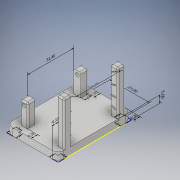
# Autodesk Inventor part: FanTable
Saved by Autodesk Inventor 2019 (Build 230136000, 136)
## iProperties
Created: 2018-06-07
Part Number: FanTable
Material: Ogólny
Document SubType Name: Modeling
Designer: Kamil
Density: 1 g/cm^3
Appearance: Domyślna
Author: Kamil
## iProperties of the stored document FanTable_Drukowanie 3D.ipt
Created: 2018-06-18
Part Number: FanTable_Drukowanie 3D
Material: Ogólny
Document SubType Name: Modeling
Designer: Kamil
Density: 1 g/cm^3
Appearance: Domyślna
Author: Kamil
Autodesk Inventor part; units mm, degrees
ref_plane "YZ Plane" through (0, 0, 0) normal (1, 0, 0) x (0, 1, 0)
ref_plane "XZ Plane" through (0, 0, 0) normal (0, 1, 0) x (-1, 0, 0)
ref_plane "XY Plane" through (0, 0, 0) normal (0, 0, 1) x (1, 0, 0)
sketch "Szkic1" plane through (0, 0, 0) normal (0, 1, 0) x (-1, 0, 0)
  line L0 (-17, -25) -> (18, -25)
  line L1 (18, -25) -> (18, 25)
  line L2 (18, 25) -> (-17, 25)
  line L3 (-17, 25) -> (-17, -25)
  dimension "d2" = 35
  dimension "d3" = 50
  constraints: 8 end point, 2 parallel, 1 horizontal, 1 perpendicular
  measures "d2" distance of L2.end L1.end
  measures "d3" distance of L1.end L0.end
extrude "Wyciągnięcie proste1" add sketch "Szkic1" along normal blind 5
sketch "Szkic2" plane through (0, 0, 0) normal (0, -1, 0) x (1, 0, 0)
  line L0 (17, 25) -> (17, -25) projected
  line L1 (17, 25) -> (13, 25)
  line L2 (13, 25) -> (13, 21)
  line L3 (13, 21) -> (17, 21)
  line L4 (17, 21) -> (17, 25)
  line L5 (-18, -25) -> (-18, 25) projected
  line L6 (-18, 25) -> (-14, 25)
  line L7 (-14, 25) -> (-14, 21)
  line L8 (-14, 21) -> (-18, 21)
  line L9 (-18, 21) -> (-18, 25)
  line L10 (17, -25) -> (-18, -25) projected
  line L11 (-18, -25) -> (-14, -25)
  line L12 (-14, -25) -> (-14, -21)
  line L13 (-14, -21) -> (-18, -21)
  line L14 (-18, -21) -> (-18, -25)
  line L15 (17, -25) -> (13, -25)
  line L16 (13, -25) -> (13, -21)
  line L17 (13, -21) -> (17, -21)
  line L18 (17, -21) -> (17, -25)
  point P0 (0, 0)
  dimension "d6" = 4
  dimension "d7" = 4
  dimension "d8" = 4
  dimension "d9" = 4
  dimension "d10" = 4
  dimension "d11" = 4
  dimension "d12" = 4
  constraints: 32 end point, 8 parallel, 4 horizontal, 4 perpendicular
  measures "d6" distance of L3.end L2.end
  measures "d7" distance of L2.end L1.end
  measures "d8" distance of L7.end L8.end
  measures "d9" distance of L6.end L7.end
  measures "d10" distance of L12.end L11.end
  measures "d11" distance of L16.end L17.end
  measures "d12" distance of L15.end L16.end
sketch "Szkic3" plane through (17, 0, 25) normal (1, 0, 0) x (0, 0, -1)
  point P0 (25, 0)
sketch "Szkic4" plane through (0, 0, 0) normal (0, -1, 0) x (1, 0, 0)
  point P0 (0, 0)
sketch "Szkic5" plane through (-18, 0, 25) normal (-1, 0, 0) x (0, 0, 1)
  point P0 (-25, 0)
fillet "Zaokrąglenie2" radius 4 1 edges at (17, 2.5, 25)
fillet "Zaokrąglenie4" radius 4 1 edges at (17, 2.5, -25)
fillet "Zaokrąglenie6" radius 4 1 edges at (-18, 2.5, 25)
fillet "Zaokrąglenie8" radius 4 1 edges at (-18, 2.5, -25)
sketch "Szkic7" plane through (0, 5, 0) normal (0, 1, 0) x (1, 0, 0)
  line L0 (-13, 15.7) -> (-8, 15.7)
  line L1 (-8, 15.7) -> (-8, 20.7)
  line L2 (-8, 20.7) -> (-13, 20.7)
  line L3 (-13, 20.7) -> (-13, 15.7)
  line L4 (-13, -15.7) -> (-8, -15.7)
  line L5 (-8, -15.7) -> (-8, -20.7)
  line L6 (-8, -20.7) -> (-13, -20.7)
  line L7 (-13, -20.7) -> (-13, -15.7)
  point P0 (0, 0)
  dimension "d114" = 1.5
  dimension "d31" = 5
  dimension "d32" = 5
  dimension "d33" = 5
  dimension "d34" = 5
  constraints: 16 end point, 4 parallel, 2 horizontal, 2 perpendicular
  measures "d31" distance of L2.end L1.end
  measures "d32" distance of L1.end L0.end
  measures "d33" distance of L5.end L6.end
  measures "d34" distance of L4.end L5.end
extrude "Wyciągnięcie proste4" add sketch "Szkic7" along normal blind 15
sketch "Szkic8" plane through (-13, 5, -15.7) normal (0, 0, 1) x (1, 0, 0)
  circle A0 centre (2.5, 12.5) radius 1.25
  point P0 (13, -5)
  dimension "d37" = 2.5
  constraints: 1 centre point
  measures "d37" diameter of A0
sketch "Szkic9" plane through (-8, 5, 15.7) normal (0, 0, -1) x (-1, 0, 0)
  circle A0 centre (2.5, 12.5) radius 1.25
  point P0 (-8, -5)
  dimension "d159" = 2.5
  constraints: 1 centre point
  measures "d159" diameter of A0
fillet "Zaokrąglenie9" radius 1 1 edges at (-13, 20, -18.2)
fillet "Zaokrąglenie10" radius 1 3 edges at (-10, 20, -20.7) (-12.7071, 19.7071, -20.7) (-13, 12, -20.7)
fillet "Zaokrąglenie11" radius 1 3 edges at (-8, 20, -17.7) (-8, 19.7071, -20.4071) (-8, 12, -20.7)
fillet "Zaokrąglenie12" radius 1 1 edges at (-13, 20, 18.2)
fillet "Zaokrąglenie13" radius 1 3 edges at (-10, 20, 20.7) (-12.7071, 19.7071, 20.7) (-13, 12, 20.7)
fillet "Zaokrąglenie14" radius 1 3 edges at (-8, 20, 17.7) (-8, 19.7071, 20.4071) (-8, 12, 20.7)
sketch "Szkic10" plane through (0, 5, 0) normal (0, 1, 0) x (1, 0, 0)
  line L0 (17, -21) -> (17, 21) projected
  line L1 (17, 15.7) -> (12, 15.7)
  line L2 (12, 15.7) -> (12, 20.7)
  line L3 (12, 20.7) -> (17, 20.7)
  line L4 (17, 20.7) -> (17, 15.7)
  line L5 (17, -15) -> (12, -15)
  line L6 (12, -15) -> (12, -20)
  line L7 (12, -20) -> (17, -20)
  line L8 (17, -20) -> (17, -15)
  point P0 (0, 0)
  dimension "d57" = 5
  dimension "d58" = 5
  dimension "d59" = 5
  dimension "d60" = 5
  constraints: 16 end point, 4 parallel, 2 horizontal, 2 perpendicular, 2 point on line
  measures "d57" distance of L2.end L3.end
  measures "d58" distance of L1.end L2.end
  measures "d59" distance of L7.end L6.end
  measures "d60" distance of L6.end L5.end
extrude "Wyciągnięcie proste7" add sketch "Szkic10" along normal blind 15 contours L1 L2 L3 L0
sketch "Szkic11" plane through (0, 5, 0) normal (0, 1, 0) x (1, 0, 0)
  line L0 (17, -21) -> (17, 21) projected
  line L1 (17, -15.7) -> (12, -15.7)
  line L2 (12, -15.7) -> (12, -20.7)
  line L3 (12, -20.7) -> (17, -20.7)
  line L4 (17, -20.7) -> (17, -15.7)
  point P0 (0, 0)
  dimension "d63" = 5
  dimension "d64" = 5
  constraints: 8 end point, 2 parallel, 1 horizontal, 1 perpendicular, 1 point on line
  measures "d63" distance of L3.end L2.end
  measures "d64" distance of L2.end L1.end
extrude "Wyciągnięcie proste8" add sketch "Szkic11" along normal blind 15
sketch "Szkic15" plane through (0, 20, 0) normal (0, 1, 0) x (1, 0, 0)
  line L0 (12, 15.7) -> (12, 20.7) projected
  line L1 (12, 20.7) -> (17, 20.7)
  line L2 (17, 20.7) -> (17, 15.7)
  line L3 (17, 15.7) -> (12, 15.7)
  line L4 (12, 15.7) -> (12, 20.7)
  line L5 (17, -20.7) -> (12, -20.7) projected
  line L6 (12, -15.7) -> (17, -15.7)
  line L7 (17, -15.7) -> (17, -20.7)
  line L8 (17, -20.7) -> (12, -20.7)
  line L9 (12, -20.7) -> (12, -15.7)
  point P0 (0, 0)
  dimension "d71" = 5
  dimension "d72" = 5
  dimension "d73" = 5
  constraints: 16 end point, 4 parallel, 2 horizontal, 2 perpendicular
  measures "d71" distance of L2.end L3.end
  measures "d72" distance of L5.start L8.end
  measures "d73" distance of L6.end L5.start
extrude "Wyciągnięcie proste9" add sketch "Szkic15" along normal blind 15
sketch "Szkic18" plane through (-13, 5, -15.7) normal (0, 0, 1) x (1, 0, 0)
  circle A0 centre (2.5, 12.5) radius 1.25 projected
  line L0 (2.5, 12.5) -> (36.3074, 21.5587)
  line L1 (2.5, 12.5) -> (37.5, 12.5) construction
  line L2 (2.5, 12.5) -> (37.5, 12.5)
  line L3 (2.5, 12.5) -> (37.5, 12.5) construction
  line L4 (2.5, 12.5) -> (36.3074, 3.4413)
  line L5 (2.5, 12.5) -> (37.5, 12.5) construction
  circle A1 centre (2.5, 12.5) radius 1.25 projected
  line L6 (2.5, 12.5) -> (32.8109, 30)
  line L7 (2.5, 12.5) -> (37.5, 12.5) construction
  line L8 (26.201, 26.1838) -> (28.799, 27.6838) construction
  line L9 (26.326, 25.9673) -> (28.924, 27.4673)
  line L10 (28.674, 27.9003) -> (26.076, 26.4003)
  arc A2 (26.076, 26.4003) -> (26.326, 25.9673) centre (26.201, 26.1838) ccw
  arc A3 (28.924, 27.4673) -> (28.674, 27.9003) centre (28.799, 27.6838) ccw
  line L11 (26.0511, 18.8105) -> (28.9489, 19.587) construction
  line L12 (26.1158, 18.569) -> (29.0136, 19.3455)
  line L13 (28.8842, 19.8284) -> (25.9864, 19.052)
  arc A4 (25.9864, 19.052) -> (26.1158, 18.569) centre (26.0511, 18.8105) ccw
  arc A5 (29.0136, 19.3455) -> (28.8842, 19.8284) centre (28.9489, 19.587) ccw
  line L14 (26, 12.5) -> (29, 12.5) construction
  line L15 (26, 12.25) -> (29, 12.25)
  line L16 (29, 12.75) -> (26, 12.75)
  arc A6 (26, 12.75) -> (26, 12.25) centre (26, 12.5) ccw
  arc A7 (29, 12.25) -> (29, 12.75) centre (29, 12.5) ccw
  line L17 (26.0511, 6.1895) -> (28.9489, 5.413) construction
  line L18 (25.9864, 5.948) -> (28.8842, 5.1716)
  line L19 (29.0136, 5.6545) -> (26.1158, 6.431)
  arc A8 (26.1158, 6.431) -> (25.9864, 5.948) centre (26.0511, 6.1895) ccw
  arc A9 (28.8842, 5.1716) -> (29.0136, 5.6545) centre (28.9489, 5.413) ccw
  point P0 (13, -5)
  point P1 (27.5, 26.9338)
  point P2 (27.5, 19.1987)
  point P3 (27.5, 12.5)
  point P4 (27.5, 5.8013)
  dimension "d84" = 35
  dimension "d85" = 15
  dimension "d86" = 35
  dimension "d87" = 0
  dimension "d88" = 35
  dimension "d89" = 15
  dimension "d90" = 35
  dimension "d91" = 30
  dimension "d116" = 1.5
  dimension "d117" = 0.5
  dimension "d118" = 1.5
  dimension "d119" = 0.5
  dimension "d120" = 1.5
  dimension "d121" = 0.5
  dimension "d122" = 1.5
  dimension "d123" = 0.5
  constraints: 48 end point, 16 point on circle, 16 tangent, 9 equal length, 8 centre point, 8 point on line, 4 horizontal, 4 midpoint
  measures "d84" distance of L0.start L0.end
  measures "d85" angle of L1 L0
  measures "d86" distance of L0.start L1.end
  measures "d87" distance between parallel lines of L2 L3
  measures "d88" distance of L0.start L4.end
  measures "d89" angle of L4 L5
  measures "d90" distance of L6.start L6.end
  measures "d91" angle of L7 L6
  measures "d116" distance of point (27.5, 26.934) L8.end
  measures "d117" diameter of A3
  measures "d118" distance of point (27.5, 19.199) L11.end
  measures "d119" diameter of A5
  measures "d120" distance of point (27.5, 12.5) L14.end
  measures "d121" diameter of A7
  measures "d122" distance of point (27.5, 5.801) L17.end
  measures "d123" diameter of A9
sketch "Szkic24" plane through (-8, 5, 15.7) normal (0, 0, -1) x (-1, 0, 0)
  circle A0 centre (2.5, 12.5) radius 1
  line L0 (2.5, 12.5) -> (-32.5, 12.5)
  line L1 (2.5, 12.5) -> (-31.3074, 21.5587) construction
  line L2 (2.5, 12.5) -> (-31.3074, 21.5587)
  line L3 (2.5, 12.5) -> (-31.3074, 21.5587) construction
  line L4 (2.5, 12.5) -> (-27.8109, 30)
  line L5 (2.5, 12.5) -> (-31.3074, 21.5587) construction
  circle A1 centre (2.5, 12.5) radius 1
  line L6 (2.5, 12.5) -> (-31.3074, 3.4413)
  line L7 (2.5, 12.5) -> (-31.3074, 21.5587) construction
  line L8 (-23.799, 27.6838) -> (-21.201, 26.1838) construction
  line L9 (-23.924, 27.4673) -> (-21.326, 25.9673)
  line L10 (-21.076, 26.4003) -> (-23.674, 27.9003)
  arc A2 (-23.674, 27.9003) -> (-23.924, 27.4673) centre (-23.799, 27.6838) ccw
  arc A3 (-21.326, 25.9673) -> (-21.076, 26.4003) centre (-21.201, 26.1838) ccw
  line L11 (-23.9489, 19.587) -> (-21.0511, 18.8105) construction
  line L12 (-24.0136, 19.3455) -> (-21.1158, 18.569)
  line L13 (-20.9864, 19.052) -> (-23.8842, 19.8284)
  arc A4 (-23.8842, 19.8284) -> (-24.0136, 19.3455) centre (-23.9489, 19.587) ccw
  arc A5 (-21.1158, 18.569) -> (-20.9864, 19.052) centre (-21.0511, 18.8105) ccw
  line L14 (-23.9353, 12.5) -> (-20.9353, 12.5) construction
  line L15 (-23.9353, 12.25) -> (-20.9353, 12.25)
  line L16 (-20.9353, 12.75) -> (-23.9353, 12.75)
  arc A6 (-23.9353, 12.75) -> (-23.9353, 12.25) centre (-23.9353, 12.5) ccw
  arc A7 (-20.9353, 12.25) -> (-20.9353, 12.75) centre (-20.9353, 12.5) ccw
  line L17 (-20.9864, 6.2068) -> (-23.8842, 5.4304) construction
  line L18 (-21.0511, 6.4483) -> (-23.9489, 5.6719)
  line L19 (-23.8195, 5.1889) -> (-20.9217, 5.9654)
  arc A8 (-20.9217, 5.9654) -> (-21.0511, 6.4483) centre (-20.9864, 6.2068) ccw
  arc A9 (-23.9489, 5.6719) -> (-23.8195, 5.1889) centre (-23.8842, 5.4304) ccw
  point P0 (-8, -5)
  point P1 (13, -2)
  point P2 (-22.5, 26.9338)
  point P3 (-22.5, 19.1987)
  point P4 (-22.4353, 12.5)
  point P5 (-22.4353, 5.8186)
  dimension "d100" = 35
  dimension "d101" = 15
  dimension "d102" = 35
  dimension "d103" = 0
  dimension "d104" = 35
  dimension "d105" = 15
  dimension "d106" = 35
  dimension "d107" = 30
  dimension "d108" = 1.5
  dimension "d109" = 0.5
  dimension "d110" = 1.5
  dimension "d111" = 0.5
  dimension "d112" = 1.5
  dimension "d113" = 0.5
  dimension "d114" = 1.5
  dimension "d115" = 0.5
  constraints: 48 end point, 16 point on circle, 16 tangent, 10 centre point, 9 equal length, 8 point on line, 4 midpoint
  measures "d100" distance of L0.start L0.end
  measures "d101" angle of L1 L0
  measures "d102" distance of L0.start L1.end
  measures "d103" distance between parallel lines of L2 L3
  measures "d104" distance of L0.start L4.end
  measures "d105" angle of L4 L5
  measures "d106" distance of L6.start L6.end
  measures "d107" angle of L7 L6
  measures "d108" distance of point (-22.5, 26.934) L8.end
  measures "d109" diameter of A3
  measures "d110" distance of point (-22.5, 19.199) L11.end
  measures "d111" diameter of A5
  measures "d112" distance of point (-22.435, 12.5) L14.end
  measures "d113" diameter of A7
  measures "d114" distance of point (-22.435, 5.819) L17.end
  measures "d115" diameter of A9
sketch "Szkic25" plane through (12, 5, -15.7) normal (0, 0, 1) x (1, 0, 0)
  point P0 (-12, -5)
extrude "Wyciągnięcie proste10" add sketch "Szkic18" along normal blind 0.5 contours A4 L13 A5 L0 | L0 A5 L12 A4 | A6 L16 A7 L2 | L2 A7 L15 A6 | A8 L19 A9 L4 | L4 A9 L18 A8 | A2 L10 A3 L6 | L6 A3 L9 A2
extrude "Wyciągnięcie proste11" add sketch "Szkic24" along normal blind 0.5 contours A7 L15 A6 L0 | L0 A6 L16 A7 | A5 L12 A4 L2 | L2 A4 L13 A5 | A3 L9 A2 L4 | L4 A2 L10 A3 | A8 L19 A9 L6 | L6 A9 L18 A8
fillet "Zaokrąglenie23" radius 1 1 edges at (14.5, 35, 20.7)
fillet "Zaokrąglenie24" radius 1 3 edges at (17, 35, 17.7) (17, 34.7071, 20.4071) (17, 19.5, 20.7)
fillet "Zaokrąglenie25" radius 1 3 edges at (12, 35, 17.7) (12, 34.7071, 20.4071) (12, 19.5, 20.7)
fillet "Zaokrąglenie26" radius 1 5 edges at (14.5, 35, 15.7) (12.2929, 34.7071, 15.7) (12, 19.5, 15.7) (16.7071, 34.7071, 15.7) (17, 19.5, 15.7)
fillet "Zaokrąglenie27" radius 1 1 edges at (14.5, 35, -15.7)
fillet "Zaokrąglenie28" radius 1 3 edges at (17, 35, -18.7) (17, 34.7071, -15.9929) (17, 19.5, -15.7)
fillet "Zaokrąglenie29" radius 1 3 edges at (12, 35, -18.7) (12, 34.7071, -15.9929) (12, 19.5, -15.7)
fillet "Zaokrąglenie30" radius 1 5 edges at (14.5, 35, -20.7) (12.2929, 34.7071, -20.7) (12, 19.5, -20.7) (16.7071, 34.7071, -20.7) (17, 19.5, -20.7)
extrude "Wyciągnięcie proste13" cut sketch "Szkic8" against normal blind 5
extrude "Wyciągnięcie proste14" cut sketch "Szkic9" against normal blind 5
